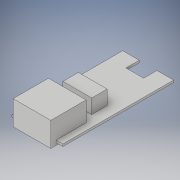
# Autodesk Inventor part: Final smaller ethernet
Saved by Autodesk Inventor 2018 (Build 220112000, 112)
## iProperties
Created: 2019-11-08
Part Number: Final smaller ethernet
Material: Generic
Document SubType Name: Modeling
Designer: Jacob
Density: 1 g/cm^3
Appearance: Default
Author: Jacob
Autodesk Inventor part; units mm, degrees
ref_plane "YZ Plane" through (0, 0, 0) normal (1, 0, 0) x (0, 1, 0)
ref_plane "XZ Plane" through (0, 0, 0) normal (0, 1, 0) x (-1, 0, 0)
ref_plane "XY Plane" through (0, 0, 0) normal (0, 0, 1) x (1, 0, 0)
sketch "Sketch1" plane through (0, 0, 0) normal (0, 1, 0) x (-1, 0, 0)
  line L0 (11.5, -25) -> (-11.5, -25)
  line L1 (-11.5, -25) -> (-11.5, 25)
  line L2 (-11.5, 25) -> (11.5, 25)
  line L3 (11.5, 25) -> (11.5, -25)
  line L4 (11.5, -25) -> (-11.5, 25) construction
  line L5 (-11.5, -25) -> (11.5, 25) construction
  point P0 (0, 0)
  dimension "d0" = 50
  dimension "d1" = 23
  constraints: 12 end point, 2 midpoint, 2 parallel, 1 horizontal, 1 perpendicular
  measures "d0" distance of L2.end L0.start
  measures "d1" distance of L0.start L0.end
extrude "Extrusion1" add sketch "Sketch1" along normal blind 1
sketch "Sketch2" plane through (0, 1, 0) normal (0, 1, 0) x (1, 0, 0)
  line L0 (-11.5, -25) -> (11.5, -25) projected
  line L1 (0, -25) -> (0, 25) construction
  line L2 (11.5, 25) -> (-11.5, 25) projected
  line L3 (-8.5, -27.5) -> (8.5, -27.5)
  line L4 (8.5, -27.5) -> (8.5, -11.5)
  line L5 (8.5, -11.5) -> (-8.5, -11.5)
  line L6 (-8.5, -11.5) -> (-8.5, -27.5)
  line L7 (-8.5, -27.5) -> (8.5, -11.5) construction
  line L8 (8.5, -27.5) -> (-8.5, -11.5) construction
  point P0 (0, 0)
  point P1 (0, -19.5)
  dimension "d4" = 2.5
  dimension "d5" = 17
  dimension "d6" = 16
  constraints: 14 end point, 4 midpoint, 2 parallel, 1 horizontal, 1 perpendicular, 1 point on line
  measures "d4" distance between parallel lines of L0 L3
  measures "d5" distance of L4.end L5.end
  measures "d6" distance of L5.end L3.start
extrude "Extrusion2" add sketch "Sketch2" along normal blind 9
sketch "Sketch3" plane through (0, 0, 0) normal (0, -1, 0) x (1, 0, 0)
  line L0 (8.5, 11.5) -> (8.5, 25) projected
  line L1 (8.5, 27.5) -> (8.5, 25) projected
  line L2 (-8.5, 27.5) -> (8.5, 27.5) projected
  line L3 (-8.5, 25) -> (-8.5, 27.5) projected
  line L4 (-8.5, 11.5) -> (8.5, 11.5) projected
  line L5 (-8.5, 25) -> (-8.5, 11.5) projected
  point P0 (0, 0)
extrude "Extrusion3" add sketch "Sketch3" along normal mid plane 2
sketch "Sketch4" plane through (0, 1, 0) normal (0, 1, 0) x (1, 0, 0)
  line L0 (8.5, -11.5) -> (-8.5, -11.5) projected
  line L1 (0, -11.5) -> (0, 25) construction
  line L2 (-11.5, 25) -> (11.5, 25) projected
  line L3 (6.5, -7) -> (-6.5, -7)
  line L4 (-6.5, -7) -> (-6.5, 0)
  line L5 (-6.5, 0) -> (6.5, 0)
  line L6 (6.5, 0) -> (6.5, -7)
  line L7 (6.5, -7) -> (-6.5, 0) construction
  line L8 (-6.5, -7) -> (6.5, 0) construction
  point P0 (0, 0)
  point P1 (0, -3.5)
  dimension "d11" = 4.5
  dimension "d12" = 7
  dimension "d13" = 13
  constraints: 14 end point, 4 midpoint, 2 parallel, 1 horizontal, 1 perpendicular, 1 point on line
  measures "d11" distance between parallel lines of L0 L3
  measures "d12" distance of L3.end L4.end
  measures "d13" distance of L4.end L5.end
extrude "Extrusion4" add sketch "Sketch4" along normal blind 6.5
sketch "Sketch5" plane through (0, 1, 0) normal (0, 1, 0) x (1, 0, 0)
  line L0 (0, 0) -> (0, 25) construction
  line L1 (11.5, 25) -> (-11.5, 25) projected
  line L2 (4, 19) -> (-4, 19)
  line L3 (-4, 19) -> (-4, 25)
  line L4 (-4, 25) -> (4, 25)
  line L5 (4, 25) -> (4, 19)
  line L6 (4, 19) -> (-4, 25) construction
  line L7 (-4, 19) -> (4, 25) construction
  point P0 (0, 22)
  dimension "d16" = 0
  dimension "d17" = 8
  dimension "d18" = 6
  constraints: 14 end point, 3 midpoint, 2 parallel, 1 horizontal, 1 perpendicular, 1 point on line
  measures "d16" distance between parallel lines of L1 L4
  measures "d17" distance of L2.start L2.end
  measures "d18" distance of L2.end L3.end
extrude "Extrusion5" cut sketch "Sketch5" against normal blind 6.5
body "Solid1"
